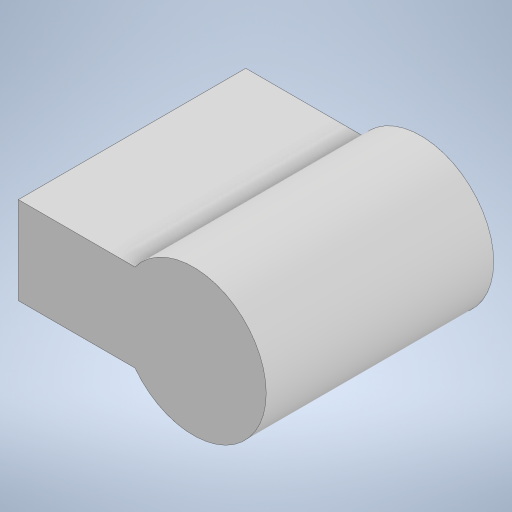
# Autodesk Inventor part: Arm 4 v0.1
Saved by Autodesk Inventor 2023 (Build 270158000, 158)
## iProperties
Created: 2024-06-24
Part Number: Arm 4 v0.1
Material: Generic
Document SubType Name: Modeling
Designer: Swoby
Density: 1 g/cm^3
Appearance: Default
Author: Swoby
Autodesk Inventor part; units mm, degrees
ref_plane "YZ Plane" through (0, 0, 0) normal (1, 0, 0) x (0, 1, 0)
ref_plane "XZ Plane" through (0, 0, 0) normal (0, 1, 0) x (-1, 0, 0)
ref_plane "XY Plane" through (0, 0, 0) normal (0, 0, 1) x (1, 0, 0)
sketch "Sketch1" plane through (0, 0, 0) normal (0, 0, 1) x (1, 0, 0)
  circle A0 centre (0, 0) radius 25
  circle A1 centre (0, 0) radius 10
  line L0 (-60, 15) -> (-20, 15)
  line L1 (-20, 15) -> (-20, -15)
  line L2 (-20, -15) -> (-60, -15)
  line L3 (-60, -15) -> (-60, 15)
  point P0 (-40, -15)
  point P1 (-20, -15)
  dimension "d0" = 50
  dimension "d1" = 20
  dimension "d2" = 30
  dimension "d3" = 15
  dimension "d4" = 40
  constraints: 8 end point, 2 coincident, 2 parallel, 1 centre point, 1 horizontal, 1 midpoint, 1 perpendicular, 3 other
  measures "d1" diameter of A1
  measures "d2" distance from line of point (-40, -15) L0
  measures "d3" distance from line of L0 point (0, 0)
  measures "d4" distance of L0.start L0.end
extrude "Extrusion1" add sketch "Sketch1" along normal mid plane 78 contours A0 L1 | L1 A0 | A0 L2 L3 L0 | A1
equation "\"d3\" = 0.5 * d2"
body "Solid1"
